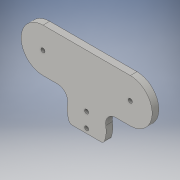
# Autodesk Inventor part: casing
Saved by Autodesk Inventor 2016 (Build 200138000, 138)
## iProperties
Created: 2019-02-22
Part Number: casing
Material: Generic
Document SubType Name: Modeling
Designer: reesem783
Density: 1 g/cm^3
Appearance: Default
Author: reesem783
Autodesk Inventor part; units mm, degrees
ref_plane "YZ Plane" through (0, 0, 0) normal (1, 0, 0) x (0, 1, 0)
ref_plane "XZ Plane" through (0, 0, 0) normal (0, 1, 0) x (-1, 0, 0)
ref_plane "XY Plane" through (0, 0, 0) normal (0, 0, 1) x (1, 0, 0)
sketch "Sketch1" plane through (0, 0, 0) normal (0, 0, 1) x (1, 0, 0)
  line L0 (0, 0) -> (76.2, 0)
  arc A0 (0, 0) -> (0, -38.1) centre (0, -19.05) ccw
  arc A1 (76.2, -38.1) -> (76.2, 0) centre (76.2, -19.05) ccw
  line L1 (76.2, -38.1) -> (63.5, -38.1)
  line L2 (0, -38.1) -> (12.7, -38.1)
  arc A2 (21.4597, -48.4605) -> (12.7, -38.1) centre (12.7, -46.9833) ccw
  arc A3 (21.4597, -48.4605) -> (22.5109, -60.7745) centre (45.8763, -52.578) ccw
  arc A4 (22.5109, -60.7745) -> (25.5069, -62.8985) centre (25.5069, -59.7235) ccw
  line L3 (25.5069, -62.8985) -> (50.6931, -62.8985)
  circle A5 centre (0, -19.05) radius 1.778
  circle A6 centre (76.2, -19.05) radius 1.778
  line L4 (-19.05, -19.05) -> (-19.05, 0)
  line L5 (95.25, -19.05) -> (95.25, 0)
  line L6 (30.3237, -52.578) -> (45.8763, -52.578)
  circle A7 centre (38.1, -46.228) radius 1.778
  circle A8 centre (38.1, -58.928) radius 1.778
  arc A9 (63.5, -38.1) -> (54.7403, -48.4605) centre (63.5, -46.9833) ccw
  arc A10 (53.6891, -60.7745) -> (54.7403, -48.4605) centre (30.3237, -52.578) ccw
  arc A11 (50.6931, -62.8985) -> (53.6891, -60.7745) centre (50.6931, -59.7235) ccw
  point P0 (23.3871, -62.9395)
  dimension "d0" = 76.2
  dimension "d1" = 38.1
  dimension "d5" = 12.7
  dimension "d6" = 12.7
  dimension "d8" = 3.175
  dimension "d9" = 3.556
  dimension "d10" = 3.556
  dimension "d14" = 19.05
  dimension "d15" = 19.05
  dimension "d16" = 3.556
  dimension "d17" = 6.35
  dimension "d18" = 3.556
  dimension "d19" = 12.7
  dimension "d22" = 6.35
  constraints: 19 point on circle, 14 end point, 12 centre point, 5 tangent, 3 horizontal, 2 coincident, 2 vertical, 1 point on line
  measures "d0" distance of L0.start L0.end
  measures "d1" distance of L0.start L2.start
  measures "d5" distance of L1.start L1.end
  measures "d6" distance of L2.start L2.end
  measures "d8" radius of A4
  measures "d9" diameter of A5
  measures "d10" diameter of A6
  measures "d14" horizontal distance of L0.start L4.start
  measures "d15" horizontal distance of L0.end L5.start
  measures "d16" diameter of A7
  measures "d17" distance from line of A7.centre L6
  measures "d18" diameter of A8
  measures "d19" distance of A7.centre A8.centre
  measures "d22" distance edge to line of A7 L2
extrude "Extrusion3" add sketch "Sketch1" along normal blind 5.842
body "Solid3"
